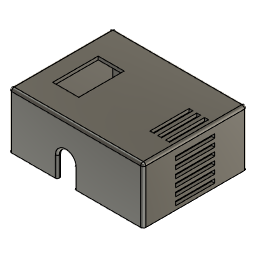
ClimbSim_Box v7 (Autodesk Fusion 360 design; units mm, degrees)
Autodesk Fusion 360 part; units mm, degrees
sketch "スケッチ1" plane through (0, 0, 0) normal (0, 0, 1) x (1, 0, 0)
  line L0 (-51.75, 40) -> (51.75, 40)
  line L1 (51.75, 40) -> (51.75, -40)
  line L2 (51.75, -40) -> (-51.75, -40)
  line L3 (-51.75, -40) -> (-51.75, 40)
  dimension "d1" = 103.5
  dimension "d2" = 80
  dimension "d32" = 51.75
  dimension "d33" = 40
  constraint horizontal L0
  constraint vertical L1
  constraint horizontal L2
  constraint vertical L3
  measures "d1" distance of L0.start L0.end
  measures "d2" distance of L0.end L1.end
  measures "d32" horizontal distance of origin L0.start
  measures "d33" vertical distance of origin L1.end
extrude "押し出し1" add sketch "スケッチ1" along normal blind 2.5 makes body 1
extrude "押し出し4" add sketch "スケッチ1" along normal blind 43 separate body makes body 2
shell "シェル2" thickness 2.5 removed faces 1 at (-17.25, -13.3333, 0) on bodies 2
sketch "スケッチ2" plane through (0, -40, 0) normal (0, -1, 0) x (1, 0, 0)
  line L0 (-51.75, 0) -> (51.75, 0)
  line L1 (51.75, 0) -> (51.75, 43)
  line L2 (51.75, 43) -> (-51.75, 43)
  line L3 (-51.75, 43) -> (-51.75, 0)
  line L4 (-14.5, 0) -> (-14.5, 15.5)
  arc A0 (-1.5, 15.5) -> (-14.5, 15.5) centre (-8, 15.5) ccw
  line L5 (-1.5, 15.5) -> (-1.5, 0)
  line L6 (-14.5, 0) -> (-1.5, 0)
  dimension "d13" = 13
  dimension "d45" = 15.5
  dimension "d46" = 8
  constraint coincident L0 L4.start
  constraint perpendicular L0 L4
  constraint tangent L4 A0
  constraint coincident L0 L5.end
  constraint tangent A0 L5
  constraint perpendicular L0 L5
  measures "d13" distance of L4.start L5.end
  measures "d45" vertical distance of origin A0.centre
  measures "d46" horizontal distance of A0.centre origin
extrude "押し出し5" cut sketch "スケッチ2" against normal blind 20 contours L0 L4 A0 L5 L6 bodies 2
sketch "スケッチ3" plane through (0, 40, 0) normal (0, 1, 0) x (-1, 0, 0)
  line L0 (-25, -15) -> (-25, 10)
  arc A0 (-15, 10) -> (-25, 10) centre (-20, 10) ccw
  line L1 (-15, 10) -> (-15, -15)
  line L2 (-15, -15) -> (-25, -15)
  line L3 (-51.75, 0) -> (51.75, 0)
  line L4 (51.75, 0) -> (51.75, 43)
  line L5 (51.75, 43) -> (-51.75, 43)
  line L6 (-51.75, 43) -> (-51.75, 0)
  dimension "d17" = 10
  dimension "d42" = 10
  dimension "d44" = 20
  constraint tangent L0 A0
  constraint tangent A0 L1
  constraint perpendicular L0 L2
  measures "d17" distance of L0.start L1.end
  measures "d42" vertical distance of A0.centre origin
  measures "d44" horizontal distance of origin A0.centre
extrude "押し出し6" cut sketch "スケッチ3" against normal blind 16 contours L0 A0 L1 L3 bodies 2
fillet "フィレット1" radius 2 4 edges at (-51.75, 40, 21.5) (51.75, 40, 21.5) (51.75, -40, 21.5) (-51.75, -40, 21.5) 1 faces at (-17.25, -13.3333, 43) on bodies 2
fillet "フィレット1" radius 1.5 6 edges at (-14.5, -40, 7.75) (-8, -40, 22) (-1.5, -40, 7.75) (25, 40, 5) (20, 40, 15) (15, 40, 5) on bodies 2
sketch "スケッチ4" plane through (0, 0, 2.5) normal (0, 0, 1) x (-1, 0, 0)
  line L0 (51.75, 40) -> (-51.75, 40)
  line L1 (-51.75, 40) -> (-51.75, -40)
  line L2 (-51.75, -40) -> (51.75, -40)
  line L3 (51.75, -40) -> (51.75, 40)
  line L4 (47.75, -36) -> (-47.75, -36)
  line L5 (-47.75, -36) -> (-47.75, 36)
  line L6 (-47.75, 36) -> (47.75, 36)
  line L7 (47.75, 36) -> (47.75, -36)
  dimension "d20" = 95.5
  dimension "d21" = 72
  dimension "d22" = 47.75
  dimension "d23" = 36
  constraint horizontal L4
  constraint vertical L5
  constraint horizontal L6
  constraint vertical L7
  measures "d20" distance of L4.start L4.end
  measures "d21" distance of L4.start L6.end
  measures "d22" horizontal distance of origin L4.start
  measures "d23" vertical distance of origin L4.start
extrude "押し出し7" add sketch "スケッチ4" along normal blind 2 contours L4 L5 L6 L7 bodies 1
sketch "スケッチ6" plane through (0, 0, 0) normal (0, 0, 1) x (1, 0, 0)
  circle A0 centre (-44.5, -32.75) radius 3
  circle A1 centre (1, -32.75) radius 3
  circle A2 centre (-44.5, 32.75) radius 3
  circle A3 centre (1, 32.75) radius 3
  circle A4 centre (6, -14.75) radius 3
  circle A5 centre (43, -14.75) radius 3
  circle A6 centre (43, 22.75) radius 3
  circle A7 centre (6, 22.75) radius 3
  circle A8 centre (-44.5, -32.75) radius 1.65
  circle A9 centre (1, -32.75) radius 1.65
  circle A10 centre (6, -14.75) radius 1.65
  circle A11 centre (43, -14.75) radius 1.65
  circle A12 centre (43, 22.75) radius 1.65
  circle A13 centre (6, 22.75) radius 1.65
  circle A14 centre (1, 32.75) radius 1.65
  circle A15 centre (-44.5, 32.75) radius 1.65
  dimension "d26" = 6
  dimension "d27" = 45.5
  dimension "d28" = 65.5
  dimension "d29" = 32.75
  dimension "d30" = 37
  dimension "d31" = 37.5
  dimension "d34" = 44.5
  dimension "d35" = 5
  dimension "d39" = 3.3
  dimension "d57" = 10
  constraint horizontal A6.centre A7.centre
  constraint vertical A4.centre A7.centre
  constraint horizontal A4.centre A5.centre
  constraint vertical A5.centre A6.centre
  constraint horizontal A0.centre A1.centre
  constraint vertical A0.centre A2.centre
  constraint horizontal A2.centre A3.centre
  constraint equal A4 A5
  constraint equal A6 A7
  constraint equal A5 A6
  constraint equal A1 A4
  constraint equal A0 A1
  constraint equal A0 A2
  constraint equal A2 A3
  constraint vertical A1.centre A3.centre
  constraint concentric A0 A8
  constraint concentric A1 A9
  constraint concentric A4 A10
  constraint concentric A5 A11
  constraint concentric A6 A12
  constraint concentric A7 A13
  constraint concentric A3 A14
  constraint concentric A2 A15
  constraint equal A8 A15
  constraint equal A8 A9
  constraint equal A9 A10
  constraint equal A10 A11
  constraint equal A11 A12
  constraint equal A12 A13
  constraint equal A13 A14
  measures "d26" diameter of A3
  measures "d27" distance of A2.centre A3.centre
  measures "d28" distance of A0.centre A2.centre
  measures "d29" vertical distance of A0.centre origin
  measures "d30" distance of A4.centre A5.centre
  measures "d31" distance of A5.centre A6.centre
  measures "d34" horizontal distance of A2.centre origin
  measures "d35" horizontal distance of A3.centre A7.centre
  measures "d39" diameter of A8
  measures "d57" vertical distance of A7.centre A3.centre
extrude "押し出し8" cut sketch "スケッチ6" along normal blind 2 contours A0 | A1 | A2 | A3 | A4 | A5 | A6 | A7 | A8 | A9 | A10 | A11 | A12 | A13 | A14 | A15 bodies 1
extrude "押し出し9" cut sketch "スケッチ6" along normal through all contours A8 | A9 | A10 | A11 | A12 | A13 | A14 | A15 bodies 1
sketch "スケッチ8" plane through (0, 0, 2.5) normal (0, 0, 1) x (-1, 0, 0)
  line L0 (-47.75, -36) -> (-47.75, 36)
  line L1 (51.75, 40) -> (-51.75, 40)
  line L2 (-51.75, 40) -> (-51.75, -40)
  line L3 (-51.75, -40) -> (51.75, -40)
  line L4 (-37, -37.25) -> (-49, -25.25)
  line L5 (-49, -37.25) -> (-37, -37.25)
  line L6 (-49, 37.25) -> (-49, 25.25)
  line L7 (-49, 25.25) -> (-37, 37.25)
  line L8 (-37, 37.25) -> (-49, 37.25)
  line L9 (-49, -37.25) -> (-49, -25.25)
  line L10 (49, -25) -> (44, -25)
  line L11 (44, -25) -> (44, 25)
  line L12 (44, 25) -> (49, 25)
  line L13 (49, 25) -> (49, -25)
  line L14 (39.5, -37.25) -> (4.5, -37.25)
  line L15 (4.5, -37.25) -> (4.5, -32.25)
  line L16 (4.5, -32.25) -> (39.5, -32.25)
  line L17 (39.5, -32.25) -> (39.5, -37.25)
  line L18 (4.5, 32.25) -> (39.5, 32.25)
  line L19 (39.5, 32.25) -> (39.5, 37.25)
  line L20 (39.5, 37.25) -> (4.5, 37.25)
  line L21 (4.5, 37.25) -> (4.5, 32.25)
  dimension "d50" = 49
  dimension "d51" = 74.5
  dimension "d52" = 37.25
  dimension "d53" = 12
  dimension "d58" = 50
  dimension "d59" = 5
  dimension "d60" = 49
  dimension "d61" = 25
  dimension "d63" = 35
  dimension "d64" = 4.5
  constraint perpendicular L6 L8
  constraint perpendicular L5 L9
  constraint equal L6 L8
  constraint equal L5 L9
  constraint equal L6 L9
  constraint vertical L4.end L6.end
  constraint vertical L9
  constraint horizontal L8
  constraint horizontal L10
  constraint vertical L11
  constraint horizontal L12
  constraint vertical L13
  constraint horizontal L14
  constraint vertical L15
  constraint horizontal L16
  constraint vertical L17
  constraint horizontal L18
  constraint vertical L19
  constraint horizontal L20
  constraint vertical L21
  constraint horizontal L7.end L20.end
  constraint horizontal L4.start L14.end
  constraint equal L15 L21
  constraint equal L10 L17
  constraint equal L16 L18
  constraint vertical L16.end L18.end
  measures "d50" horizontal distance of origin L6.start
  measures "d51" distance of L5.start L6.start
  measures "d52" vertical distance of origin L5.start
  measures "d53" horizontal distance of L5.start L4.start
  measures "d58" distance of L10.start L12.end
  measures "d59" distance of L10.start L10.end
  measures "d60" horizontal distance of origin L12.end
  measures "d61" vertical distance of origin L12.end
  measures "d63" distance of L14.start L14.end
  measures "d64" horizontal distance of origin L15.end
extrude "押し出し10" add sketch "スケッチ8" along normal blind 5 bodies 1
fillet "フィレット2" radius 2 4 edges at (-51.75, -40, 1.25) (51.75, -40, 1.25) (51.75, 40, 1.25) (-51.75, 40, 1.25) on bodies 1
sketch "スケッチ10" plane through (0, 0, 43) normal (0, 0, 1) x (-1, 0, 0)
  line L0 (49.75, 38) -> (-49.75, 38)
  line L1 (-49.75, 38) -> (-49.75, -38)
  line L2 (-49.75, -38) -> (49.75, -38)
  line L3 (49.75, -38) -> (49.75, 38)
  line L4 (38, -15) -> (18, -15)
  line L5 (18, -15) -> (18, 20)
  line L6 (18, 20) -> (38, 20)
  line L7 (38, 20) -> (38, -15)
  dimension "d73" = 15
  dimension "d74" = 20
  dimension "d75" = 18
  dimension "d76" = 20
  constraint horizontal L4
  constraint vertical L5
  constraint horizontal L6
  constraint vertical L7
  measures "d73" vertical distance of origin L4.end
  measures "d74" vertical distance of origin L5.end
  measures "d75" horizontal distance of origin L5.end
  measures "d76" distance of L5.end L6.end
extrude "押し出し13" cut sketch "スケッチ10" against normal blind 25 contours L4 L5 L6 L7 bodies 2
sketch "スケッチ9" plane through (51.75, 0, 0) normal (1, 0, 0) x (0, 1, 0)
  line L0 (-38, 41) -> (-38, 0)
  line L1 (-38, 0) -> (38, 0)
  line L2 (38, 0) -> (38, 41)
  line L3 (38, 41) -> (-38, 41)
  line L4 (-15, 36) -> (15, 36)
  line L5 (15, 36) -> (15, 33)
  line L6 (15, 33) -> (-15, 33)
  line L7 (-15, 33) -> (-15, 36)
  line L8 (15, 27) -> (-15, 27)
  line L9 (-15, 30) -> (15, 30)
  line L10 (15, 30) -> (15, 27)
  line L11 (-15, 27) -> (-15, 30)
  line L12 (15, 21) -> (-15, 21)
  line L13 (-15, 24) -> (15, 24)
  line L14 (15, 24) -> (15, 21)
  line L15 (-15, 21) -> (-15, 24)
  line L16 (15, 15) -> (-15, 15)
  line L17 (-15, 18) -> (15, 18)
  line L18 (15, 18) -> (15, 15)
  line L19 (-15, 15) -> (-15, 18)
  line L20 (15, 9) -> (-15, 9)
  line L21 (-15, 12) -> (15, 12)
  line L22 (15, 12) -> (15, 9)
  line L23 (-15, 9) -> (-15, 12)
  line L24 (15, 3) -> (-15, 3)
  line L25 (-15, 6) -> (15, 6)
  line L26 (15, 6) -> (15, 3)
  line L27 (-15, 3) -> (-15, 6)
  dimension "d80" = 30
  dimension "d81" = 3
  dimension "d82" = 15
  dimension "d85" = 0
  dimension "d86" = -6
  dimension "d89" = 36
  constraint horizontal L4
  constraint vertical L5
  constraint horizontal L6
  constraint vertical L7
  measures "d80" distance of L4.start L4.end
  measures "d81" distance of L4.end L5.end
  measures "d82" horizontal distance of origin L6.end
  measures "d89" vertical distance of origin L4.start
extrude "押し出し14" cut sketch "スケッチ9" against normal blind 10 contours L4 L5 L6 L7 | L8 L9 L10 L11 | L12 L13 L14 L15 | L16 L17 L18 L19 | L20 L21 L22 L23 | L24 L25 L26 L27 bodies 2
sketch "スケッチ11" plane through (0, 0, 43) normal (0, 0, 1) x (-1, 0, 0)
  line L0 (18, -15) -> (18, 20)
  line L1 (18, 20) -> (38, 20)
  line L2 (38, 20) -> (38, -15)
  line L3 (38, -15) -> (18, -15)
  line L4 (49.75, 38) -> (-49.75, 38)
  line L5 (-49.75, 38) -> (-49.75, -38)
  line L6 (-49.75, -38) -> (49.75, -38)
  line L7 (49.75, -38) -> (49.75, 38)
  line L8 (-47, -15) -> (-44, -15)
  line L9 (-44, -15) -> (-44, 15)
  line L10 (-44, 15) -> (-47, 15)
  line L11 (-47, 15) -> (-47, -15)
  line L12 (-41, -15) -> (-38, -15)
  line L13 (-38, -15) -> (-38, 15)
  line L14 (-38, 15) -> (-41, 15)
  line L15 (-41, 15) -> (-41, -15)
  line L16 (-35, -15) -> (-32, -15)
  line L17 (-32, -15) -> (-32, 15)
  line L18 (-32, 15) -> (-35, 15)
  line L19 (-35, 15) -> (-35, -15)
  dimension "d90" = 3
  dimension "d91" = 30
  dimension "d92" = 15
  constraint horizontal L8
  constraint vertical L9
  constraint horizontal L10
  constraint vertical L11
  constraint horizontal L12
  constraint vertical L13
  constraint horizontal L14
  constraint vertical L15
  constraint horizontal L16
  constraint vertical L17
  constraint horizontal L18
  constraint vertical L19
  constraint equal L14 L18
  constraint equal L10 L14
  constraint equal L9 L13
  constraint equal L13 L17
  measures "d90" distance of L9.end L10.end
  measures "d91" distance of L8.start L10.end
  measures "d92" vertical distance of origin L10.end
extrude "押し出し15" cut sketch "スケッチ11" against normal blind 20 contours L8 L9 L10 L11 | L12 L13 L14 L15 | L16 L17 L18 L19 bodies 2
hidden bodies 1
equation "d1 = 93.5 mm + 10 mm"
equation "d22 = ( 95.5 / 2 ) * 1 mm"
equation "d28 = 70 mm - 4.5 mm"
equation "d29 = ( 65.5 / 2 ) * 1 mm"
equation "d30 = 43.5 mm - 6.5 mm"
equation "d32 = ( 103.5 / 2 ) * 1 mm"
